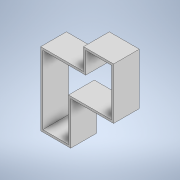
# Autodesk Inventor part: s_room
Saved by Autodesk Inventor 2022 (Build 260153000, 153)
## iProperties
Created: 2022-10-21
Part Number: s_room
Material: Generic
Document SubType Name: Modeling
Designer: Matthew
Density: 1 g/cm^3
Appearance: Default
Author: Matthew
Autodesk Inventor part; units mm, degrees
ref_plane "YZ Plane" through (0, 0, 0) normal (1, 0, 0) x (0, 1, 0)
ref_plane "XZ Plane" through (0, 0, 0) normal (0, 1, 0) x (-1, 0, 0)
ref_plane "XY Plane" through (0, 0, 0) normal (0, 0, 1) x (1, 0, 0)
sketch "Sketch1" plane through (0, 0, 0) normal (0, 0, 1) x (1, 0, 0)
  line L0 (0, 0) -> (152.4, 0)
  line L1 (152.4, 0) -> (152.4, 254)
  line L2 (0, 254) -> (0, 0)
  line L3 (152.4, 254) -> (406.4, 254)
  line L4 (406.4, 254) -> (406.4, 406.4)
  line L5 (254, 406.4) -> (0, 406.4)
  line L6 (0, 406.4) -> (0, 254)
  line L7 (254, 406.4) -> (254, 533.4)
  line L8 (254, 533.4) -> (406.4, 533.4)
  line L9 (406.4, 533.4) -> (406.4, 406.4)
  line L10 (-12.7, 419.1) -> (241.3, 419.1)
  line L11 (241.3, 419.1) -> (241.3, 546.1)
  line L12 (241.3, 546.1) -> (419.1, 546.1)
  line L13 (419.1, 546.1) -> (419.1, 406.4)
  line L14 (419.1, 406.4) -> (419.1, 241.3)
  line L15 (419.1, 241.3) -> (165.1, 241.3)
  line L16 (165.1, 241.3) -> (165.1, -12.7)
  line L17 (165.1, -12.7) -> (-12.7, -12.7)
  line L18 (-12.7, -12.7) -> (-12.7, 254)
  line L19 (-12.7, 254) -> (-12.7, 419.1)
  dimension "d6" = 12.7
  constraints: 40 end point, 8 parallel, 4 perpendicular, 2 horizontal, 9 other
  measures "d6" distance between parallel lines of L5 L10
extrude "Extrusion1" add sketch "Sketch1" along normal blind 152.4
body "Solid1"
